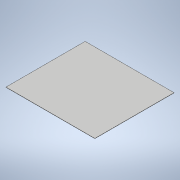
# Autodesk Inventor part: seatfloor
Saved by Autodesk Inventor 2021 (Build 250183000, 183)
## iProperties
Created: 2020-10-26
Part Number: seatfloor
Material: Generic
Document SubType Name: Modeling
Designer: mackeycj
Density: 1 g/cm^3
Appearance: Default
Author: mackeycj
Autodesk Inventor part; units mm, degrees
ref_plane "YZ Plane" through (0, 0, 0) normal (1, 0, 0) x (0, 1, 0)
ref_plane "XZ Plane" through (0, 0, 0) normal (0, 1, 0) x (-1, 0, 0)
ref_plane "XY Plane" through (0, 0, 0) normal (0, 0, 1) x (1, 0, 0)
sketch "Sketch1" plane through (0, 0, 0) normal (0, 1, 0) x (-1, 0, 0)
  line L0 (-279.4, -248.92) -> (279.4, -248.92)
  line L1 (279.4, -248.92) -> (279.4, 248.92)
  line L2 (279.4, 248.92) -> (-279.4, 248.92)
  line L3 (-279.4, 248.92) -> (-279.4, -248.92)
  line L4 (-279.4, -248.92) -> (279.4, 248.92) construction
  line L5 (279.4, -248.92) -> (-279.4, 248.92) construction
  point P0 (0, 0)
  dimension "d0" = 558.8
  dimension "d1" = 497.84
  constraints: 12 end point, 2 midpoint, 2 parallel, 1 horizontal, 1 perpendicular
  measures "d0" distance of L2.end L1.end
  measures "d1" distance of L1.end L0.end
extrude "Extrusion1" add sketch "Sketch1" along normal blind 1.524
body "Solid1"
